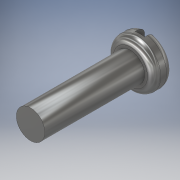
# Autodesk Inventor part: Schraube
Saved by Autodesk Inventor 2017 SP1 (Build 210196100, 196)
## iProperties
Part Number: Schraube
Material: Generisch
Document SubType Name: Modeling
Designer: Alex
Density: 1 g/cm^3
Appearance: Vorgabe
Author: Alex
Autodesk Inventor part; units mm, degrees
ref_plane "YZ Plane" through (0, 0, 0) normal (1, 0, 0) x (0, 1, 0)
ref_plane "XZ Plane" through (0, 0, 0) normal (0, 1, 0) x (-1, 0, 0)
ref_plane "XY Plane" through (0, 0, 0) normal (0, 0, 1) x (1, 0, 0)
sketch "Skizze1" plane through (0, 0, 0) normal (0, 1, 0) x (-1, 0, 0)
  circle A0 centre (0, 0) radius 2.5
  dimension "d0" = 5
  constraints: 1 centre point, 1 coincident
  measures "d0" diameter of A0
extrude "Extrusion1" add sketch "Skizze1" along normal blind 2
sketch "Skizze2" plane through (0, 2, 0) normal (0, 1, 0) x (1, 0, 0)
  line L0 (-0.5, -3.2562) -> (0.5, -3.2562)
  line L1 (0.5, -3.2562) -> (0.5, 3.274)
  line L2 (0.5, 3.274) -> (-0.5, 3.274)
  line L3 (-0.5, 3.274) -> (-0.5, -3.2562)
  line L4 (1.5, -0.5) -> (-1.5, -0.5)
  line L5 (-1.5, -0.5) -> (-1.5, 0.5)
  line L6 (-1.5, 0.5) -> (1.5, 0.5)
  line L7 (1.5, 0.5) -> (1.5, -0.5)
  point P0 (0, 0)
  dimension "d3" = 1
  dimension "d4" = 1
  dimension "d5" = 0.5
  dimension "d6" = 0.5
  dimension "d7" = 3
  dimension "d8" = 1.5
  constraints: 16 end point, 4 parallel, 2 horizontal, 2 perpendicular
  measures "d3" distance between parallel lines of L1 L3
  measures "d4" distance of L6.end L4.start
  measures "d5" distance from line of L1 point (0, 0)
  measures "d6" distance from line of point (0, 0) L4
  measures "d7" distance of L5.end L6.end
  measures "d8" distance from line of L7 point (0, 0)
fillet "Rundung1" radius 0.7 2 edges at (2.5, 2, 0) (2.5, 0, 0)
extrude "Extrusion2" cut sketch "Skizze2" against normal blind 1
sketch "Skizze3" plane through (0, 0, 0) normal (0, -1, 0) x (1, 0, 0)
  circle A0 centre (0, 0) radius 1.5
  dimension "d12" = 3
  constraints: 1 centre point, 1 coincident
  measures "d12" diameter of A0
extrude "Extrusion3" add sketch "Skizze3" along normal blind 10.5
